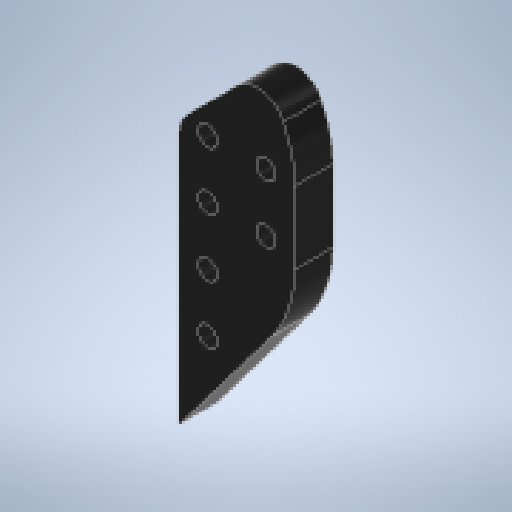
# Autodesk Inventor part: IntakeArmSpacingBlock
Saved by Autodesk Inventor 2023 (Build 270158000, 158)
## iProperties
Created: 2022-11-11
Part Number: IntakeArmSpacingBlock
Material: ABS Plastic
Document SubType Name: Modeling
Designer: Zac Hah
Density: 1.06 g/cm^3
Appearance: Smooth - Black
Author: Zac Hah
Autodesk Inventor part; units mm, degrees
ref_plane "YZ Plane" through (0, 0, 0) normal (1, 0, 0) x (0, 1, 0)
ref_plane "XZ Plane" through (0, 0, 0) normal (0, 1, 0) x (-1, 0, 0)
sketch "Sketch1" plane through (0, 0, 0) normal (0, 0, 1) x (1, 0, 0)
  arc A0 (1.9234, 26.2171) -> (0.0635, 21.727) centre (6.4135, 21.727) ccw projected
  line L0 (0.0635, 21.727) -> (0.0635, 10.6083) projected
  arc A1 (-1.2167, 6.7848) -> (0.0635, 10.6083) centre (-6.2865, 10.6083) ccw projected
  line L1 (-1.2167, 6.7848) -> (-22.9032, -21.9707) projected
  arc A2 (-22.9032, -21.9707) -> (-2.6238, -37.2648) centre (-12.7635, -29.6178) ccw projected
  line L2 (-2.6238, -37.2648) -> (20.3429, -6.8118) projected
  arc A3 (20.3429, -6.8118) -> (25.4635, 8.4822) centre (0.0635, 8.4822) ccw projected
  line L3 (25.4635, 8.4822) -> (25.4635, 24.3572) projected
  arc A4 (25.4635, 24.3572) -> (22.9837, 35.3037) centre (0.0635, 24.3572) ccw projected
  arc A5 (22.9837, 35.3037) -> (12.7635, 37.0572) centre (17.2536, 32.5671) ccw projected
  line L4 (12.7635, 37.0572) -> (1.9234, 26.2171) projected
  circle A6 centre (19.1135, 24.3572) radius 2.159 projected
  circle A7 centre (6.4135, 24.3572) radius 2.159 projected
  circle A8 centre (6.4135, -13.7428) radius 2.159 projected
  circle A9 centre (6.4135, -1.0428) radius 2.159 projected
  circle A10 centre (6.4135, 11.6572) radius 2.159 projected
  circle A11 centre (19.1135, 11.6572) radius 2.159 projected
  circle A12 centre (-12.7635, -29.6178) radius 2.159 projected
  line L5 (0.0635, 10.6083) -> (0.0635, -33.7015)
  point P0 (0, 0)
  constraints: 2 end point, 1 point on line, 1 vertical
ref_plane "Work Plane1" through (-25.4635, -42.3178, 8.382) normal (0, 0, -1) x (0, 1, 0)
extrude "Extrusion1" add sketch "Sketch1" along normal up to surface (8.382 mm away) contours L4 A5 A4 L3 A3 L2 L5 L0 A0
fillet "Fillet1" radius 3.175 1 edges at (0.0635, -33.7015, 4.191)
body "Solid1"
